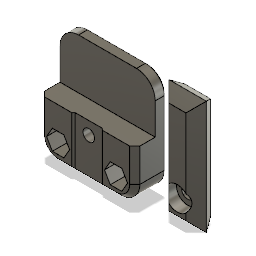
_bed low clamps.cf029c22-a421-43ba-9290-03b6b70f7262 (Autodesk Fusion 360 design; units mm, degrees)
Autodesk Fusion 360 part; units mm, degrees
note: some values were not read from the file. Chosen so that the rebuilt part matches the saved one: which face or edge a step refers to. Set by a fixed rule: which sketch regions a step uses.
sketch "Sketch1" plane through (0, 0, 0) normal (0, 0, 1) x (1, 0, 0)
  circle A0 centre (-8.5, 0) radius 1.7
  circle A1 centre (8.5, 0) radius 1.7
  circle A2 centre (0, 6) radius 1.7
  line L0 (-8.5, -5.5) -> (8.5, -5.5)
  line L1 (-14, 0) -> (-14, 18.9807)
  line L2 (-8.5, 24.4807) -> (8.5, 24.4807)
  line L3 (14, 18.9807) -> (14, 0)
  arc A3 (-8.5, 24.4807) -> (-14, 18.9807) centre (-8.5, 18.9807) ccw
  arc A4 (-14, 0) -> (-8.5, -5.5) centre (-8.5, 0) ccw
  arc A5 (8.5, -5.5) -> (14, 0) centre (8.5, 0) ccw
  arc A6 (14, 18.9807) -> (8.5, 24.4807) centre (8.5, 18.9807) ccw
  dimension "d1" = 8.5
  dimension "d2" = 8.5
  dimension "d3" = 3.4
  dimension "d4" = 3.4
  dimension "d5" = 6
  dimension "d6" = 3.4
  dimension "d7" = 11
  dimension "d8" = 11
  dimension "d11" = 11
  dimension "d12" = 11
  constraint concentric A0 A4
  constraint concentric A1 A5
  constraint tangent L0 A5
  constraint tangent L0 A4
  constraint tangent L1 A3
  constraint tangent L2 A6
  constraint tangent L3 A5
  constraint tangent L3 A6
  constraint tangent L2 A3
  constraint tangent L1 A4
  measures "d1" distance of origin A0.centre
  measures "d2" distance of origin A1.centre
  measures "d3" diameter of A0
  measures "d4" diameter of A1
  measures "d5" distance of origin A2.centre
  measures "d6" diameter of A2
  measures "d7" diameter of A4
  measures "d8" diameter of A5
  measures "d11" diameter of A6
  measures "d12" diameter of A3
extrude "Extrude1" add sketch "Sketch1" along normal blind 3.175 makes body 1
sketch "Sketch2" plane through (0, 0, 3.175) normal (0, 0, 1) x (1, 0, 0)
  circle A0 centre (0, 6) radius 1.7
  circle A1 centre (8.5, 0) radius 1.7
  circle A2 centre (-8.5, 0) radius 1.7
  arc A3 (-14, 0) -> (-8.5, -5.5) centre (-8.5, 0) ccw
  line L0 (-8.5, -5.5) -> (8.5, -5.5)
  arc A4 (8.5, -5.5) -> (14, 0) centre (8.5, 0) ccw
  line L1 (14, 0) -> (14, 18.9807)
  arc A5 (14, 18.9807) -> (8.5, 24.4807) centre (8.5, 18.9807) ccw
  line L2 (8.5, 24.4807) -> (-8.5, 24.4807)
  arc A6 (-8.5, 24.4807) -> (-14, 18.9807) centre (-8.5, 18.9807) ccw
  line L3 (-14, 18.9807) -> (-14, 0)
  line L4 (-8.5, 0) -> (-8.5, 13)
  line L5 (-14, 9.75) -> (14.0002, 9.75)
  line L6 (-5.125, 0) -> (-6.8125, 2.9228)
  line L7 (-6.8125, 2.9228) -> (-10.1875, 2.9228)
  line L8 (-10.1875, 2.9228) -> (-11.875, 0)
  line L9 (-11.875, 0) -> (-10.1875, -2.9228)
  line L10 (-10.1875, -2.9228) -> (-6.8125, -2.9228)
  line L11 (-6.8125, -2.9228) -> (-5.125, 0)
  line L12 (5.125, 0) -> (6.8125, -2.9228)
  line L13 (6.8125, -2.9228) -> (10.1875, -2.9228)
  line L14 (10.1875, -2.9228) -> (11.875, 0)
  line L15 (11.875, 0) -> (10.1875, 2.9228)
  line L16 (10.1875, 2.9228) -> (6.8125, 2.9228)
  line L17 (6.8125, 2.9228) -> (5.125, 0)
  point P0 (-8.5, 0)
  point P1 (8.5, 0)
  dimension "d15" = 13
  dimension "d16" = 3.375
  dimension "d17" = 3.375
  dimension "d51" = 15.25
  constraint coincident P0 A2.centre
  constraint vertical L4
  constraint horizontal L5
  constraint coincident L3 L5.start
  constraint coincident P1 A1.centre
  measures "d15" distance of P0 L4.end
  measures "d16" distance of L6.start P0
  measures "d17" distance of L12.start P1
  measures "d51" distance of L0 L5
extrude "Extrude2" add sketch "Sketch2" along normal blind 6 contours A3 L0 A4 L1 L3 L5 bodies 1
chamfer "Chamfer1" distance 1.5 angle 45 5 edges at (-14, 4.875, 9.175) (-12.3891, -3.8891, 9.175) (0, -5.5, 9.175) (12.3891, -3.8891, 9.175) (14, 4.875, 9.175) on bodies 1
sketch "Sketch3" plane through (0, 0, 0) normal (0, 0, -1) x (-1, 0, 0)
  circle A0 centre (8.5, 0) radius 1.7
  circle A1 centre (0, 6) radius 1.7
  circle A2 centre (-8.5, 0) radius 1.7
  arc A3 (8.5, -5.5) -> (14, 0) centre (8.5, 0) ccw
  line L0 (14, 0) -> (14, 18.9807)
  arc A4 (14, 18.9807) -> (8.5, 24.4807) centre (8.5, 18.9807) ccw
  line L1 (8.5, 24.4807) -> (-8.5, 24.4807)
  arc A5 (-8.5, 24.4807) -> (-14, 18.9807) centre (-8.5, 18.9807) ccw
  line L2 (-14, 18.9807) -> (-14, 0)
  arc A6 (-14, 0) -> (-8.5, -5.5) centre (-8.5, 0) ccw
  line L3 (-8.5, -5.5) -> (8.5, -5.5)
  line L4 (0, 2.625) -> (2.9228, 4.3125)
  line L5 (2.9228, 4.3125) -> (2.9228, 7.6875)
  line L6 (2.9228, 7.6875) -> (0, 9.375)
  line L7 (0, 9.375) -> (-2.9228, 7.6875)
  line L8 (-2.9228, 7.6875) -> (-2.9228, 4.3125)
  line L9 (-2.9228, 4.3125) -> (0, 2.625)
  point P0 (0, 6)
  dimension "d21" = 3.375
  constraint coincident P0 A1.centre
  measures "d21" distance of L4.start P0
extrude "Extrude3" cut sketch "Sketch3" against normal blind 6 contours L4 L5 L6 L7 L8 L9 bodies 1
chamfer "Chamfer2" distance 0.5 angle 45 8 edges at (14, 9.4904, 0) (12.3891, 22.8698, 0) (0, 24.4807, 0) (-12.3891, 22.8698, 0) (-14, 9.4904, 0) (-12.3891, -3.8891, 0) (0, -5.5, 0) (12.3891, -3.8891, 0) on bodies 1
chamfer "Chamfer3" distance 0.5 angle 45 8 edges at (-1.4614, 3.4688, 0) (1.4614, 3.4688, 0) (2.9228, 6, 0) (1.4614, 8.5313, 0) (-1.4614, 8.5312, 0) (-2.9228, 6, 0) (-10.085, 0.6147, 0) (6.915, 0.6147, 0) on bodies 1
sketch "Sketch4" plane through (0, 0, 9.175) normal (0, 0, 1) x (1, 0, 0)
  line L0 (-12.5, 9.75) -> (-12.5, 0)
  arc A0 (-12.5, 0) -> (-8.5, -4) centre (-8.5, 0) ccw
  line L1 (-8.5, -4) -> (8.5, -4)
  arc A1 (8.5, -4) -> (12.5, 0) centre (8.5, 0) ccw
  line L2 (12.5, 0) -> (12.5, 9.75)
  line L3 (12.5, 9.75) -> (-12.5, 9.75)
  circle A2 centre (0, 6) radius 1.7
  line L4 (-5.125, 0) -> (-6.8125, -2.9228)
  line L5 (-6.8125, -2.9228) -> (-10.1875, -2.9228)
  line L6 (-10.1875, -2.9228) -> (-11.875, 0)
  line L7 (-11.875, 0) -> (-10.1875, 2.9228)
  line L8 (-10.1875, 2.9228) -> (-6.8125, 2.9228)
  line L9 (-6.8125, 2.9228) -> (-5.125, 0)
  line L10 (5.125, 0) -> (6.8125, 2.9228)
  line L11 (6.8125, 2.9228) -> (10.1875, 2.9228)
  line L12 (10.1875, 2.9228) -> (11.875, 0)
  line L13 (11.875, 0) -> (10.1875, -2.9228)
  line L14 (10.1875, -2.9228) -> (6.8125, -2.9228)
  line L15 (6.8125, -2.9228) -> (5.125, 0)
  line L16 (4, -9) -> (-4, -9)
  line L17 (-4, -9) -> (-4, 21)
  line L18 (-4, 21) -> (4, 21)
  line L19 (4, 21) -> (4, -9)
  line L20 (4, -9) -> (-4, 21) construction
  line L21 (-4, -9) -> (4, 21) construction
  point P0 (0, 6)
  dimension "d26" = 30
  dimension "d27" = 8
  constraint perpendicular L16 L17
  constraint parallel L16 L18
  constraint parallel L17 L19
  constraint horizontal L16
  constraint coincident L20 P0
  constraint coincident L21 P0
  constraint coincident P0 A2.centre
  measures "d26" distance of L16.end L17.end
  measures "d27" distance of L17.end L18.end
extrude "Extrude4" cut sketch "Sketch4" against normal blind 0.5 contours L3 L17 L18 L19 | L1 L3 L17 L19 | L1 L16 L17 L19 | A2 bodies 1
chamfer "Chamfer4" distance 0.5 angle 45 2 edges at (4, 2.875, 9.175) (-4, 2.875, 9.175) on bodies 1
sketch "Sketch5" plane through (0, 0, 0) normal (0, 0, 1) x (1, 0, 0)
  line L0 (19.5, -5.5) -> (27.1, -5.5)
  line L1 (27.1, -5.5) -> (27.1, 24.5)
  line L2 (27.1, 24.5) -> (19.5, 24.5)
  line L3 (19.5, 24.5) -> (19.5, -5.5)
  line L4 (23.3, -5.5) -> (23.3, 2)
  circle A0 centre (23.3, 2) radius 1.7
  dimension "d31" = 30
  dimension "d32" = 7.6
  dimension "d33" = 7.5
  dimension "d34" = 3.4
  constraint horizontal L0
  constraint vertical L1
  constraint horizontal L2
  constraint vertical L3
  constraint midpoint L0 L4.start
  constraint perpendicular L0 L4
  constraint coincident L4.end A0.centre
  measures "d31" distance of L0.start L2.end
  measures "d32" distance of L0.start L0.end
  measures "d33" distance of L4.start L4.end
  measures "d34" diameter of A0
extrude "Extrude5" add sketch "Sketch5" along normal blind 3 draft 30 separate body makes body 2
delete_face "DeleteFace1" 2 faces at (22.5437, 2.5415, 1.3333) (23.4214, 1.0778, 1.3333) on bodies 2
sketch "Sketch6" plane through (0, 0, 3) normal (0, 0, 1) x (1, 0, 0)
  line L0 (28.8321, 26.2321) -> (17.7679, 26.2321)
  line L1 (17.7679, 26.2321) -> (17.7679, -7.2321)
  line L2 (17.7679, -7.2321) -> (28.8321, -7.2321)
  line L3 (28.8321, -7.2321) -> (28.8321, 26.2321)
  line L4 (23.3, -7.2321) -> (23.3, 0.2679)
  dimension "d37" = 7.5
  constraint midpoint L2 L4.start
  constraint perpendicular L2 L4
  measures "d37" distance of L4.start L4.end
extrude "Extrude6" add sketch "Sketch6" along normal blind 3 draft -45 bodies 2
sketch "Sketch7" plane through (0, 0, 3) normal (0, 0, 1) x (1, 0, 0)
  circle A0 centre (23.3, 0.2679) radius 3.75
  circle A1 centre (23.3, 0.2679) radius 1.7
  dimension "d41" = 3.4
  constraint concentric A0 A1
  measures "d41" diameter of A1
sketch "Sketch8" plane through (0, 0, 6) normal (0, 0, 1) x (1, 0, 0)
  line L0 (20.7679, -4.2321) -> (25.8321, -4.2321)
  line L1 (25.8321, -4.2321) -> (25.8321, 23.2321)
  line L2 (25.8321, 23.2321) -> (20.7679, 23.2321)
  line L3 (20.7679, 23.2321) -> (20.7679, -4.2321)
  line L4 (28.8321, -7.2321) -> (17.7679, -7.2321)
  line L5 (23.3, -7.2321) -> (23.3, 0.2679)
  circle A0 centre (23.3, 0.2679) radius 1.7
  dimension "d44" = 7.5
  dimension "d45" = 3.4
  constraint midpoint L4 L5.start
  constraint perpendicular L0 L5
  constraint coincident L5.end A0.centre
  measures "d44" distance of L5.start L5.end
  measures "d45" diameter of A0
extrude "Extrude8" cut sketch "Sketch8" against normal blind 7 contours A0 bodies 2
sketch "Sketch9" plane through (0, 0, 6) normal (0, 0, 1) x (1, 0, 0)
  circle A0 centre (23.3, 0.2679) radius 1.7
  line L0 (20.7679, -4.2321) -> (25.8321, -4.2321)
  line L1 (25.8321, -4.2321) -> (25.8321, 23.2321)
  line L2 (25.8321, 23.2321) -> (20.7679, 23.2321)
  line L3 (20.7679, 23.2321) -> (20.7679, -4.2321)
  circle A1 centre (23.3, 0.2679) radius 3.5
  dimension "d48" = 7
  constraint concentric A0 A1
  measures "d48" diameter of A1
extrude "Extrude9" cut sketch "Sketch9" against normal blind 3 draft -5 contours L3 A1 | L1 L3 A1 | L1 A1 bodies 2
delete_face "DeleteFace2" 1 faces at (24.2594, -1.3937, 3.5) on bodies 2
equation "d1 = ( 17 / 2 ) * 1 mm"
equation "d2 = ( 17 / 2 ) * 1 mm"
equation "d13 = ( 25.4 / 8 ) * 1 mm"
equation "d16 = ( 6.75 / 2 ) * 1 mm"
